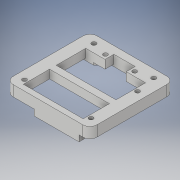
# Autodesk Inventor part: front-cam
Saved by Autodesk Inventor 2019 (Build 230136000, 136)
## iProperties
Created: 2019-02-22
Part Number: front-cam
Material: Generic
Document SubType Name: Modeling
Designer: Tesler
Density: 1 g/cm^3
Appearance: Default
Author: Tesler
Autodesk Inventor part; units mm, degrees
ref_plane "YZ Plane" through (0, 0, 0) normal (1, 0, 0) x (0, 1, 0)
ref_plane "XZ Plane" through (0, 0, 0) normal (0, 1, 0) x (-1, 0, 0)
ref_plane "XY Plane" through (0, 0, 0) normal (0, 0, 1) x (1, 0, 0)
sketch "Sketch1" plane through (0, 0, 0) normal (0, 1, 0) x (-1, 0, 0)
  line L0 (21.324, 10.54) -> (-21.324, 10.54)
  line L1 (-21.324, -33.91) -> (-15.724, -33.91)
  circle A0 centre (-23.749, -25.782) radius 1.524
  circle A1 centre (-23.749, 7.365) radius 1.524
  circle A2 centre (23.749, 7.365) radius 1.524
  circle A3 centre (10.414, -37.085) radius 1.524
  circle A4 centre (-10.414, -37.085) radius 1.524
  line L2 (-29.924, 14.3694) -> (-29.924, -45.6306)
  line L3 (29.924, 14.3694) -> (29.924, -45.6306)
  line L4 (-29.924, 14.3694) -> (29.924, 14.3694)
  line L5 (-21.324, -33.91) -> (-7.574, -33.91)
  line L6 (-7.574, -33.91) -> (-7.574, -40.26)
  line L7 (-7.574, -40.26) -> (7.574, -40.26)
  line L8 (29.924, -45.6306) -> (-29.924, -45.6306)
  line L9 (-21.324, 10.54) -> (21.324, 10.54)
  circle A5 centre (-23.749, 7.365) radius 1.524
  circle A6 centre (23.749, 7.365) radius 1.524
  circle A7 centre (-23.749, -25.782) radius 1.524
  circle A8 centre (10.414, -37.085) radius 1.524
  circle A9 centre (-10.414, -37.085) radius 1.524
  line L10 (-21.324, -8.1306) -> (21.324, -8.1306)
  line L11 (-21.324, -12.8806) -> (21.324, -12.8806)
  line L12 (-21.324, 10.54) -> (-21.324, -8.1306)
  line L13 (-21.324, -12.8806) -> (-21.324, -33.91)
  line L14 (21.324, -33.91) -> (21.324, -12.8806)
  line L15 (21.324, -8.1306) -> (21.324, 10.54)
  line L16 (21.324, -33.91) -> (7.574, -33.91)
  line L17 (7.574, -33.91) -> (7.574, -40.26)
  point P0 (0, 0)
  point P1 (-14.449, -33.91)
  dimension "d6" = 60
  dimension "d9" = 13.75
  dimension "d11" = 56.1706
  dimension "d12" = 37.5
  dimension "d13" = 32.75
  dimension "d14" = 51.248
  dimension "d15" = 8.6
  constraints: 36 end point, 10 centre point, 10 vertical, 6 perpendicular, 5 coincident, 5 concentric, 5 horizontal, 2 point on line, 1 collinear, 1 midpoint, 1 parallel, 7 other
  measures "d6" distance of L2.start L2.end
  measures "d9" distance of L1.start L5.end
  measures "d11" distance between parallel lines of L8 L0
  measures "d12" distance between parallel lines of L8 L10
  measures "d13" distance between parallel lines of L8 L11
  measures "d14" distance between parallel lines of L15 L2
  measures "d15" distance between parallel lines of L12 L2
extrude "Extrusion1" add sketch "Sketch1" along normal blind 7.62
sketch "Sketch2" plane through (0, 0, 0) normal (0, -1, 0) x (1, 0, 0)
  line L0 (21.324, 10.54) -> (-21.324, 10.54) projected
  line L1 (0, 10.54) -> (-26.924, 10.54)
  line L2 (-26.924, 10.54) -> (-26.924, -40.26)
  line L3 (-26.924, -40.26) -> (26.924, -40.26)
  line L4 (26.924, -40.26) -> (26.924, 10.54)
  line L5 (26.924, 10.54) -> (0, 10.54)
  point P0 (0, 0)
  dimension "d18" = 26.924
  dimension "d19" = 50.8
  dimension "d20" = 53.848
  constraints: 10 end point, 4 perpendicular, 1 collinear, 1 midpoint, 1 point on line
  measures "d18" distance of L1.start L1.end
  measures "d19" distance of L1.end L2.end
  measures "d20" distance of L2.end L3.end
extrude "Extrusion2" cut sketch "Sketch2" against normal blind 1.5875
fillet "Fillet1" radius 5.08 4 edges at (29.924, 3.81, 14.3694) (-29.924, 3.81, 14.3694) (29.924, 3.81, -45.6306) (-29.924, 3.81, -45.6306)
sketch "Sketch3" plane through (0, 0, 0) normal (0, -1, 0) x (1, 0, 0)
  line L0 (-24.844, 14.3694) -> (24.844, 14.3694) projected
  line L1 (-9.9342, 14.3694) -> (-9.9342, 10.54)
  line L2 (-29.924, -40.5506) -> (-29.924, 9.2894) projected
  line L3 (22.177, 14.3694) -> (22.177, 10.54)
  line L4 (-26.924, 10.54) -> (26.924, 10.54) projected
  line L5 (29.924, 9.2894) -> (29.924, -40.5506) projected
  line L6 (-9.9342, 14.3694) -> (22.177, 14.3694)
  line L7 (22.177, 10.54) -> (-9.9342, 10.54)
  point P0 (0, 0)
  dimension "d24" = 19.9898
  dimension "d25" = 7.747
  constraints: 8 end point, 3 point on line, 2 collinear, 2 vertical
  measures "d24" distance between parallel lines of L1 L2
  measures "d25" distance between parallel lines of L5 L3
extrude "Extrusion3" add sketch "Sketch3" along normal blind 4.2926
sketch "Sketch4" plane through (0, 1.5875, 0) normal (0, -1, 0) x (1, 0, 0)
  line L0 (21.324, -33.91) -> (21.324, -12.8806) projected
  line L1 (26.924, -40.26) -> (-26.924, -40.26) projected
  line L2 (-21.324, -33.91) -> (-7.574, -33.91) projected
  line L3 (-26.924, -40.26) -> (-14.224, -40.26)
  line L4 (-15.7226, -33.91) -> (-26.924, -33.91)
  line L5 (-26.924, -33.91) -> (-26.924, -40.26)
  line L6 (7.574, -33.91) -> (21.324, -33.91) projected
  line L7 (26.924, -40.26) -> (14.224, -40.26)
  line L8 (15.7226, -33.91) -> (26.924, -33.91)
  line L9 (26.924, -33.91) -> (26.924, -40.26)
  line L10 (-14.224, -40.26) -> (-14.224, -35.4086)
  circle A0 centre (-10.414, -37.085) radius 1.524 projected
  line L11 (-15.7226, -33.91) -> (-14.224, -35.4086)
  line L12 (14.224, -40.26) -> (14.224, -35.4086)
  circle A1 centre (10.414, -37.085) radius 1.524 projected
  line L13 (14.224, -35.4086) -> (15.7226, -33.91)
  point P0 (0, 0)
  dimension "d42" = 11.2014
  dimension "d43" = 11.2014
  dimension "d44" = 4.8514
  dimension "d45" = 3.81
  dimension "d46" = 4.8514
  dimension "d48" = 3.81
  dimension "d49" = 6.35
  dimension "d50" = 6.35
  constraints: 20 end point, 4 point on line, 2 horizontal, 2 parallel, 2 vertical, 1 collinear
  measures "d42" distance of L4.end L4.start
  measures "d43" distance of L8.start L8.end
  measures "d44" distance of L3.end L10.end
  measures "d45" distance from line of A0.centre L10
  measures "d46" distance of L7.end L12.end
  measures "d48" distance from line of L12 A1.centre
  measures "d49" distance of L8.end L1.start
  measures "d50" distance of L4.end L1.end
extrude "Extrusion4" add sketch "Sketch4" along normal blind 1.5875 contours L1 L5 L4 L2 L11 L10 | L1 L12 L13 L6 L8 L9
sketch "Sketch5" plane through (0, 0, 0) normal (0, -1, 0) x (1, 0, 0)
  line L0 (-14.224, -40.26) -> (-14.224, -35.4086) projected
  line L1 (-15.7226, -33.91) -> (-26.924, -33.91) projected
  line L2 (-26.924, -33.91) -> (-26.924, 10.54) projected
  line L3 (0, -57.6306) -> (0, 26.3694) projected
  line L4 (-26.924, 10.54) -> (-9.9342, 10.54) projected
  line L5 (-24.844, 14.3694) -> (-9.9342, 14.3694) projected
  line L6 (-29.924, -40.5506) -> (-29.924, 9.2894) projected
  circle A0 centre (-21.3233, -39.7647) radius 1.5875
  circle A1 centre (21.3233, -39.7647) radius 1.5875
  point P0 (0, 0)
  dimension "d101" = 3.175
  dimension "d102" = 5.8547
  dimension "d104" = 7.0993
  constraints: 2 centre point, 1 symmetric about line, 1 other
  measures "d101" diameter of A0
  measures "d102" distance from line of L1 A0.centre
  measures "d104" distance from line of L0 A0.centre
extrude "Extrusion6" cut sketch "Sketch5" against normal up to next
body "Solid1"
